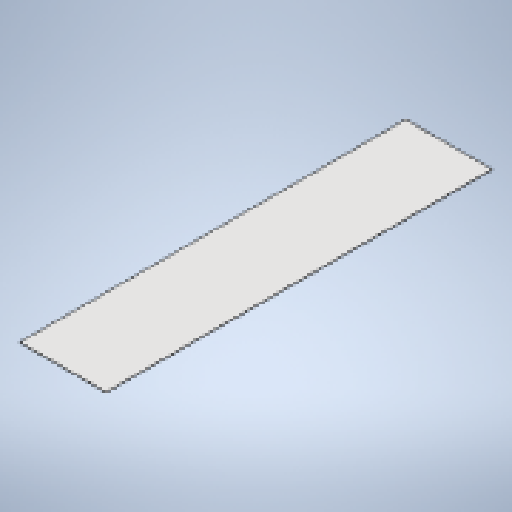
# Autodesk Inventor part: GnG frame 2 floor sheet 10
Saved by Autodesk Inventor 2025.3 (Build 293356030, 356C)
## iProperties
Created: 2025-10-28
Part Number: GnG frame 2 floor sheet 10
Material: Stainless Steel
Document SubType Name: Sheet Metal
Designer: admin
Mass: 280.619 g
Surface Area: 364.406 cm^2
Volume: 35.0774 cm^3
Density: 8 g/cm^3
Sheet Metal Rule: AISI304 3mm Die 32
Sheet Metal Width: 300,000 mm
Sheet Metal Length: 2300,000 mm
Sheet Metal Area: 690000,000 mm^2
Appearance: Default
Flat Pattern Width: 30 cm
Flat Pattern Length: 230 cm
Flat Pattern Area: 6900 cm^2
Author: admin
Autodesk Inventor part; units mm, degrees
ref_plane "YZ Plane" through (0, 0, 0) normal (1, 0, 0) x (0, 1, 0)
ref_plane "XZ Plane" through (0, 0, 0) normal (0, 1, 0) x (-1, 0, 0)
ref_plane "XY Plane" through (0, 0, 0) normal (0, 0, 1) x (1, 0, 0)
sketch "Sketch1" plane through (0, 0, 0) normal (0, 0, 1) x (1, 0, 0)
  line L0 (0, 0) -> (-300, 0)
  line L1 (-300, 0) -> (-300, -2300)
  line L2 (-300, -2300) -> (0, -2300)
  line L3 (0, -2300) -> (0, 0)
  line L4 (0, 0) -> (-40, 0)
  line L5 (-40, 0) -> (-40, -35)
  line L6 (-40, -35) -> (0, -35)
  line L7 (0, -35) -> (0, 0)
  line L8 (0, -2300) -> (-40, -2300)
  line L9 (-40, -2300) -> (-40, -2265)
  line L10 (-40, -2265) -> (0, -2265)
  line L11 (0, -2265) -> (0, -2300)
  line L12 (-300, 0) -> (-260, 0)
  line L13 (-260, 0) -> (-260, -35)
  line L14 (-260, -35) -> (-300, -35)
  line L15 (-300, -35) -> (-300, 0)
  line L16 (-300, -2300) -> (-260, -2300)
  line L17 (-260, -2300) -> (-260, -2265)
  line L18 (-260, -2265) -> (-300, -2265)
  line L19 (-300, -2265) -> (-300, -2300)
  line L20 (-240, -2300) -> (-140, -2300)
  line L21 (-140, -2300) -> (-140, -2265)
  line L22 (-140, -2265) -> (-240, -2265)
  line L23 (-240, -2265) -> (-240, -2300)
  line L24 (-240, 0) -> (-140, 0)
  line L25 (-140, 0) -> (-140, -35)
  line L26 (-140, -35) -> (-240, -35)
  line L27 (-240, -35) -> (-240, 0)
  point P0 (0, -35)
  point P1 (-40, 0)
  point P2 (0, -2265)
  point P3 (-140, -2300)
  point P4 (-140, 0)
  point P5 (-260, 0)
  point P6 (-300, -35)
  point P7 (-300, -2265)
  point P8 (-260, -2300)
  point P9 (-300, -35)
  point P10 (-300, 0)
  point P11 (-260, -2265)
  point P12 (-260, -2300)
  point P13 (-260, -35)
  point P14 (-260, 0)
  point P15 (-300, -2265)
  point P16 (-240, -2300)
  point P17 (-240, 0)
  dimension "d22" = 300
  dimension "d23" = 2300
  dimension "d24" = 40
  dimension "d25" = 35
  dimension "d28" = 100
  dimension "d29" = 100
  measures "d22" distance of L2.end L1.end
  measures "d23" distance of L1.end L0.end
  measures "d24" distance of L6.end L5.end
  measures "d25" distance of L5.end L4.end
  measures "d28" distance of L25.end L26.end
  measures "d29" distance between parallel lines of L5 L25
extrude "Plate1" add sketch "Sketch1" along normal blind 3
sketch "Sketch5" plane through (0, 0, 0) normal (0, 0, -1) x (-1, 0, 0)
  line L0 (300, 0) -> (200, 0) construction
  line L1 (200, 0) -> (200, -2) construction
  line L2 (200, -2) -> (300, -2) construction
  line L3 (300, -2) -> (300, 0) construction
  line L4 (200, 0) -> (198.4752, -4.6556)
  arc A0 (197.5248, -4.6556) -> (198.4752, -4.6556) centre (198, -4.5) ccw
  line L5 (197.5248, -4.6556) -> (196, 0)
  line L6 (196, 0) -> (200, 0)
  line L7 (196, 0) -> (194, 0) construction
  line L8 (194, 0) -> (192, 0)
  line L9 (192, 0) -> (192, -5)
  line L10 (192, -5) -> (194, -5)
  line L11 (194, -5) -> (194, 0)
  line L12 (192, 0) -> (190, 0) construction
  line L13 (190, 0) -> (188, 0)
  line L14 (188, 0) -> (188, -5)
  line L15 (188, -5) -> (190, -5)
  line L16 (190, -5) -> (190, 0)
  line L17 (188, 0) -> (186, 0) construction
  line L18 (186, 0) -> (184, 0)
  line L19 (184, 0) -> (184, -5)
  line L20 (184, -5) -> (186, -5)
  line L21 (186, -5) -> (186, 0)
  line L22 (184, 0) -> (182, 0) construction
  line L23 (182, 0) -> (180, 0)
  line L24 (180, 0) -> (180, -5)
  line L25 (180, -5) -> (182, -5)
  line L26 (182, -5) -> (182, 0)
  line L27 (180, 0) -> (175, 0) construction
  line L28 (175, 0) -> (170, 0) construction
  circle A1 centre (175, 0) radius 1
  circle A2 centre (170, 0) radius 1
  point P0 (0, 0)
  point P1 (198, 0)
  dimension "d30" = 100
  dimension "d31" = 2
  dimension "d32" = 5
  dimension "d33" = 4
  dimension "d34" = 0.5
  dimension "d35" = 5
  dimension "d36" = 5
  dimension "d37" = 5
  dimension "d38" = 2
  constraints: 58 end point, 11 horizontal, 10 equal length, 10 parallel, 5 perpendicular, 4 coincident, 3 centre point, 3 tangent, 2 point on circle, 1 equal radius, 1 midpoint, 1 point on line, 1 vertical alignment
  measures "d30" distance of L2.end L1.end
  measures "d31" distance of L1.end L0.end
  measures "d32" distance of L9.end L9.start
  measures "d33" distance of L5.end L0.end
  measures "d34" radius of A0
  measures "d35" distance of L15.start L13.end
  measures "d36" distance of L19.end L19.start
  measures "d37" distance of L24.end L24.start
  measures "d38" diameter of A1
extrude "Cut1" cut sketch "Sketch5" against normal blind 3 contours L26 L25 L24 L23 | A1 | A2
sketch "Sketch6" plane through (0, 0, 0) normal (0, 0, -1) x (-1, 0, 0)
  circle A0 centre (194.6369, -998.5751) radius 19.7563
  point P0 (0, 0)
  constraints: 1 centre point
extrude "Cut2" cut sketch "Sketch6" against normal blind 3
equation "\"d33\" = 2 * d31"
equation "\"d34\" = 0.25 * d31"
equation "\"d38\" = d31"
equation "\"d39\" = Thickness"
equation "\"d41\" = Thickness"
equation "\"d2\" = Thickness"
equation "\"BendReliefWidth\" = Thickness"
equation "\"BendReliefDepth\" = 0.5 * Thickness"
equation "\"CornerReliefSize\" = 4 * Thickness"
equation "\"MinimumRemnant\" = 2 * Thickness"
equation "\"TransitionRadius\" = BendRadius"
equation "\"JacobiRadiusSize\" = BendRadius"
equation "\"GapSize\" = Thickness"
equation "\"Thickness\" = 3"
equation "\"BendRadius\" = 5"
body "Solid1"
